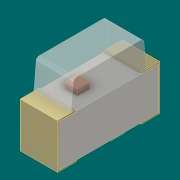
# Autodesk Inventor part: LTST-S270GKT
Saved by Autodesk Inventor 2016 SP2 (Build 200236200, 236)
## iProperties
Created: 2016-05-25
Part Number: LTST-S270GKT
Material: ABS Plastic
Document SubType Name: Modeling
Designer: Sawaiz
Density: 1.06 g/cm^3
Appearance: Smooth - White
Author: Sawaiz
Autodesk Inventor part; units mm, degrees
ref_plane "YZ Plane" through (0, 0, 0) normal (1, 0, 0) x (0, 1, 0)
ref_plane "XZ Plane" through (0, 0, 0) normal (0, 1, 0) x (-1, 0, 0)
ref_plane "XY Plane" through (0, 0, 0) normal (0, 0, 1) x (1, 0, 0)
sketch "Sketch1" plane through (0, 0, 0) normal (0, 0, 1) x (1, 0, 0)
  line L0 (0.8, 0.3) -> (-0.8, 0.3)
  line L1 (-0.8, 0.3) -> (-0.8, -0.3)
  line L2 (-0.8, -0.3) -> (0.8, -0.3)
  line L3 (0.8, -0.3) -> (0.8, 0.3)
  line L4 (0.8, 0.3) -> (-0.8, -0.3) construction
  line L5 (-0.8, 0.3) -> (0.8, -0.3) construction
  point P0 (0, 0)
  dimension "d0" = 1.6
  dimension "d1" = 0.6
  constraints: 12 end point, 2 midpoint, 2 parallel, 1 horizontal, 1 perpendicular
  measures "d0" distance of L2.end L1.end
  measures "d1" distance of L1.end L0.end
extrude "Extrusion1" add sketch "Sketch1" along normal blind 0.68
sketch "Sketch2" plane through (0, 0, 0.68) normal (0, 0, 1) x (1, 0, 0)
  line L0 (0.8, 0.3) -> (-0.8, 0.3) projected
  line L1 (-0.8, 0.3) -> (-0.8, -0.3) projected
  line L2 (-0.8, -0.3) -> (0.8, -0.3) projected
  line L3 (0.8, -0.3) -> (0.8, 0.3) projected
  line L4 (0.3, 0.1) -> (0.1, 0.1)
  line L5 (0.1, 0.1) -> (0.1, -0.1)
  line L6 (0.1, -0.1) -> (0.3, -0.1)
  line L7 (0.3, -0.1) -> (0.3, 0.1)
  line L8 (0.3, 0.1) -> (0.1, -0.1) construction
  line L9 (0.1, 0.1) -> (0.3, -0.1) construction
  point P0 (0, 0)
  point P1 (0.2, 0)
  dimension "d4" = 0.2
  dimension "d5" = 0.2
  dimension "d6" = 1
  constraints: 12 end point, 2 midpoint, 2 parallel, 1 horizontal, 1 perpendicular
  measures "d4" distance of L6.end L5.end
  measures "d5" distance of L5.end L4.end
  measures "d6" distance from line of L1 point (0.2, 0)
extrude "Extrusion2" add sketch "Sketch2" along normal blind 0.1 separate body contours L7 L6 L5 L4
sketch "Sketch3" plane through (-0.8, 0.3, 0) normal (0, 1, 0) x (1, 0, 0)
  line L0 (1.6, 0) -> (0, 0) projected
  line L1 (0, 0) -> (0, -0.68) projected
  line L2 (1.6, -0.68) -> (0, -0.68) projected
  line L3 (1.6, 0) -> (1.6, -0.68) projected
  line L4 (1.32, -0.68) -> (1.32, -0.7)
  line L5 (1.32, -0.7) -> (1.62, -0.7)
  line L6 (1.62, -0.7) -> (1.62, 0.02)
  line L7 (1.62, 0.02) -> (1.32, 0.02)
  line L8 (1.32, 0.02) -> (1.32, 0)
  line L9 (1.6, 0) -> (0, 0) projected
  point P0 (0.8, 0)
  dimension "d9" = 0.02
  dimension "d10" = 0.02
  dimension "d11" = 0.02
  dimension "d12" = 0.3
  constraints: 10 end point, 4 point on line, 2 perpendicular, 1 parallel, 1 vertical
  measures "d9" distance between parallel lines of L2 L5
  measures "d10" distance between parallel lines of L0 L7
  measures "d11" distance between parallel lines of L6 L3
  measures "d12" distance between parallel lines of L6 L4
extrude "Extrusion3" add sketch "Sketch3" against normal up to surface (0.6 mm away) separate body contours L0 L8 L7 L6 L5 L4 L2 L3
mirror "Mirror1" about plane through (0, 0, 0) normal (1, 0, 0) of "Extrusion3" bodies 3
sketch "Sketch4" plane through (0, 0, 0.68) normal (0, 0, 1) x (1, 0, 0)
  line L0 (0.8, 0.3) -> (-0.8, 0.3) projected
  line L1 (-0.8, 0.3) -> (-0.8, -0.3) projected
  line L2 (-0.8, -0.3) -> (0.8, -0.3) projected
  line L3 (0.8, -0.3) -> (0.8, 0.3) projected
  line L4 (0.6123, 0.3) -> (-0.6123, 0.3)
  line L5 (-0.6123, 0.3) -> (-0.6123, -0.3)
  line L6 (-0.6123, -0.3) -> (0.6123, -0.3)
  line L7 (0.6123, -0.3) -> (0.6123, 0.3)
  line L8 (0.6123, 0.3) -> (-0.6123, -0.3) construction
  line L9 (-0.6123, 0.3) -> (0.6123, -0.3) construction
  line L10 (0.52, 0.3) -> (0.52, -0.3) projected
  line L11 (-0.52, 0.3) -> (-0.52, -0.3) projected
  point P0 (0, 0)
  constraints: 12 end point, 2 midpoint, 2 parallel, 1 horizontal, 1 perpendicular, 1 point on line
extrude "Extrusion4" add sketch "Sketch4" along normal up to surface (0.02 mm away) separate body contours L10 L2 L11 L0
sketch "Sketch5" plane through (-0.52, 0.3, 0.7) normal (0, 0, 1) x (1, 0, 0)
  line L0 (1.04, 0) -> (1.04, -0.6) projected
  line L1 (0, 0) -> (1.04, 0) projected
  line L2 (0, -0.6) -> (0, 0) projected
  line L3 (1.04, -0.6) -> (0, -0.6) projected
  line L4 (1.12, 0) -> (-0.08, 0)
  line L5 (-0.08, 0) -> (-0.08, -0.6)
  line L6 (-0.08, -0.6) -> (1.12, -0.6)
  line L7 (1.12, -0.6) -> (1.12, 0)
  line L8 (1.12, 0) -> (-0.08, -0.6) construction
  line L9 (-0.08, 0) -> (1.12, -0.6) construction
  point P0 (0.52, -0.3)
  dimension "d17" = 1.2
  constraints: 12 end point, 2 midpoint, 2 parallel, 1 horizontal, 1 perpendicular
  measures "d17" distance of L6.end L5.end
extrude "Extrusion5" add sketch "Sketch5" along normal blind 0.45 bodies 4
sketch "Sketch6" plane through (-0.52, 0.3, 0.68) normal (0, 1, 0) x (1, 0, 0)
  line L0 (1.04, 0) -> (1.04, -0.02) projected
  line L1 (1.04, 0) -> (0, 0) projected
  line L2 (0, 0) -> (0, -0.02) projected
  line L3 (0, -0.02) -> (-0.08, -0.02) projected
  line L4 (-0.08, -0.02) -> (-0.08, -0.47) projected
  line L5 (1.12, -0.47) -> (-0.08, -0.47) projected
  line L6 (1.12, -0.02) -> (1.12, -0.47) projected
  line L7 (1.12, -0.02) -> (1.04, -0.02) projected
  line L8 (1.12, -0.02) -> (1.0806, -0.47)
  line L9 (-0.08, -0.02) -> (-0.0406, -0.47)
  point P0 (0.52, 0.68)
  dimension "d20" = 5
  dimension "d21" = 5
  constraints: 4 end point, 2 point on line
  measures "d20" angle of L6 L8
  measures "d21" angle of L4 L9
extrude "Extrusion6" cut sketch "Sketch6" against normal through all contours L6 L5 L8 | L9 L5 L4 bodies 4
fillet "Fillet1" radius 0.05 2 edges at (0.5606, 0, 1.15) (-0.5606, 0, 1.15)
sketch "Sketch7" plane through (0, 0, 0) normal (0, 0, -1) x (-1, 0, 0)
  line L0 (-0.8, 0.3) -> (0.8, 0.3) projected
  line L1 (-0.8, -0.3) -> (-0.8, 0.3) projected
  line L2 (0.8, -0.3) -> (-0.8, -0.3) projected
  line L3 (0.8, 0.3) -> (0.8, -0.3) projected
  line L4 (-0.8, 0.3) -> (0.8, 0.3) projected
  line L5 (0.25, -0.3) -> (0.05, -0.3)
  line L6 (0.05, -0.3) -> (0.05, 0.3)
  line L7 (0.05, 0.3) -> (0.25, 0.3)
  line L8 (0.25, 0.3) -> (0.25, -0.3)
  line L9 (0.25, -0.3) -> (0.05, 0.3) construction
  line L10 (0.05, -0.3) -> (0.25, 0.3) construction
  line L11 (0.05, -0.1) -> (-0.15, -0.1)
  line L12 (-0.15, -0.1) -> (-0.15, 0.1)
  line L13 (-0.15, 0.1) -> (0.05, 0.1)
  line L14 (0.05, 0.1) -> (0.05, -0.1)
  line L15 (0.8, -0.3) -> (-0.8, -0.3) projected
  point P0 (0, 0)
  point P1 (0.15, 0)
  dimension "d25" = 0.1
  dimension "d26" = 0.1
  dimension "d27" = 0.2
  dimension "d28" = 0.05
  dimension "d29" = 0.15
  constraints: 20 end point, 4 parallel, 2 horizontal, 2 midpoint, 2 perpendicular, 2 point on line, 1 collinear
  measures "d25" distance from line of point (0, 0) L11
  measures "d26" distance from line of L13 point (0, 0)
  measures "d27" distance between parallel lines of L8 L6
  measures "d28" distance from line of point (0, 0) L6
  measures "d29" distance from line of point (0, 0) L12
extrude "Extrusion7" add sketch "Sketch7" along normal blind 0.01 separate body contours L0 L8 L2 L6 | L6 L11 L12 L13
equation "\"d21\" = d20"
body "Solid1"
body "Solid2"
body "Solid3"
body "Solid4"
body "Solid5"
